Autodesk Fusion 360 part; units mm, degrees
(part 3 of 3)
extrude "Extrusion26" cut sketch "Skizze19" along normal blind 0.5 from surface at -2 contours L26 L27 L30 L31 L32 L33 | L28 L29 L34 L35 L36 L37 bodies 2
chamfer "Fase6" distance 0.2 angle 45 4 edges at (0.75, 45.5, -31) (2, 47.75, -31) (0.75, 4, -31) (2, 1.75, -31) on bodies 2
sketch "Skizze20" plane through (0, 0, -31.5) normal (0, 0, 1) x (-1, 0, 0)
  line L0 (-2, -50) -> (0.5, -50)
  line L1 (0.5, -50) -> (0.5, -45.5)
  line L2 (0.5, -45.5) -> (-2, -45.5)
  line L3 (-2, -45.5) -> (-2, -50)
  line L4 (-2, 0.5) -> (-2, -4)
  line L5 (-2, -4) -> (0.5, -4)
  line L6 (0.5, -4) -> (0.5, 0.5)
  line L7 (0.5, 0.5) -> (-2, 0.5)
  line L8 (0.35, -45.65) -> (-1.85, -45.65)
  line L9 (-1.85, -45.65) -> (-1.85, -49.85)
  line L10 (-1.85, -49.85) -> (0.35, -49.85)
  line L11 (0.35, -49.85) -> (0.35, -45.65)
  line L12 (0.35, 0.35) -> (-1.85, 0.35)
  line L13 (-1.85, 0.35) -> (-1.85, -3.85)
  line L14 (-1.85, -3.85) -> (0.35, -3.85)
  line L15 (0.35, -3.85) -> (0.35, 0.35)
  dimension "d117" = -0.15
  dimension "d118" = -0.15
extrude "Extrusion27" add sketch "Skizze20" along normal blind 27.7 separate body contours L12 L13 L14 L15 makes body 6
extrude "Extrusion28" add sketch "Skizze20" along normal blind 27.7 separate body contours L8 L9 L10 L11 makes body 7
extrude "Extrusion29" add 1 faces at (73.55, 39, -18.6167) along direction (0, -1, 0) blind 3 on bodies 5 bodies 5
sketch "Skizze21" plane through (0, 0, -33) normal (0, 0, -1) x (1, 0, 0)
  line L0 (75.9, -1.1) -> (1.1, -1.1)
  line L1 (75.9, -48.4) -> (75.9, -1.1)
  line L2 (1.1, -48.4) -> (75.9, -48.4)
  line L3 (2.5, -45) -> (2.5, -50)
  line L4 (2.5, -50) -> (2.5, -45)
  line L5 (-0.5, -45) -> (2.5, -45)
  line L6 (2.5, -45) -> (-0.5, -45)
  line L7 (1.1, -1.1) -> (1.1, -48.4)
  line L8 (2.5, -4.5) -> (-0.5, -4.5)
  line L9 (2.5, 0.5) -> (2.5, -4.5)
  line L10 (2.5, -4.5) -> (2.5, 0.5)
  line L11 (-0.4, 0.4) -> (-0.4, -49.9)
  line L12 (-0.4, -49.9) -> (77.4, -49.9)
  line L13 (77.4, 0.4) -> (77.4, -49.9)
  line L14 (77.4, 0.4) -> (-0.4, 0.4)
  line L15 (1.1, -1.1) -> (4, -1.1)
  line L16 (1.1, -6) -> (1.1, -1.1)
  line L17 (-0.4, -49.9) -> (4, -49.9)
  line L18 (4, -49.9) -> (4, -43.5)
  line L19 (4, -43.5) -> (-0.4, -43.5)
  line L20 (-0.4, -43.5) -> (-0.4, -49.9)
  line L21 (-0.5, 0.5) -> (4, 0.5)
  line L22 (4, 0.5) -> (4, -5.9931)
  line L23 (4, -5.9931) -> (-0.5, -5.9931)
  line L24 (-0.5, -5.9931) -> (-0.5, 0.5)
  line L25 (1.1, -6.4786) -> (4.3748, -6.4786)
  line L26 (4.3748, -6.4786) -> (4.3748, -1.1)
  line L27 (1.1, -6.4786) -> (1.1, -1.1)
  point P0 (-0.5, 0.5)
  dimension "d121" = 2.9
  dimension "d122" = 4.9
  dimension "d123" = 4.4
  dimension "d124" = 6.4
  constraint horizontal L15
  constraint vertical L16
  constraint coincident L0.end L7.start
  constraint horizontal L17
  constraint vertical L18
  constraint horizontal L19
  constraint vertical L20
  constraint coincident L11.end L12.start
  constraint horizontal L21
  constraint vertical L22
  constraint horizontal L23
  constraint vertical L24
  constraint coincident P0 L21.start
  constraint coincident L7 L25.start
  constraint perpendicular L7 L25
  constraint coincident L0 L26.end
  constraint perpendicular L0 L26
  measures "d121" distance of L0.end L15.end
  measures "d122" distance of L0.end L16.start
  measures "d123" distance of L11.end L17.end
  measures "d124" distance of L11.end L19.end
extrude "Extrusion30" add sketch "Skizze21" against normal blind 3 contours L0 L1 L2 L12 L13 L14 L18 L22 | L0 L7 L8 L9 L10 L15 L16 L22 L23 L27 | L0 L9 L10 L14 L15 L22 | L2 L3 L4 L12 L17 L18 | L2 L3 L4 L5 L6 L7 L18 L19 | L7 L11 L16 L19 L23 L27 | L7 L8 L11 L16 L23 L27 | L5 L6 L7 L11 L19 L20 bodies 4
equation "d29 = 3.5 mm + 1.6 mm - 0.5 mm"
equation "d33 = d32 / 2"
equation "d91 = -1.50 mm - 10 mm - 1 mm"
equation "d121 = 1.400 mm + 1.5 mm"
equation "d122 = 3.400 mm + 1.5 mm"
equation "d123 = 2.900 mm + 1.5 mm"
equation "d124 = 4.900 mm + 1.5 mm"
named bodies: "Print", "Case_MK2", "Backplate_MK2", "Lid_MK2", "ResetBtn_MK2", "Holder1_MK2", "Holder2_MK2"
